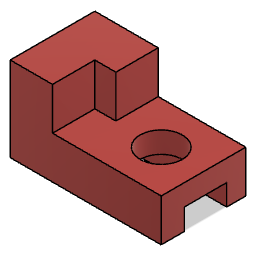
3d14 v1 (Autodesk Fusion 360 design; units mm, degrees)
Autodesk Fusion 360 part; units mm, degrees
sketch "Sketch1" plane through (0, 0, 0) normal (0, 0, 1) x (1, 0, 0)
  line L0 (0, 0) -> (0, 28)
  line L1 (0, 28) -> (14, 28)
  line L2 (14, 28) -> (14, 14)
  line L3 (14, 14) -> (50, 14)
  line L4 (50, 14) -> (50, 0)
  line L5 (50, 0) -> (0, 0)
  dimension "d1" = 14
  dimension "d2" = 14
  dimension "d3" = 14
  dimension "d4" = 50
  constraint coincident L0.start L5.end
  constraint vertical L0
  constraint perpendicular L0 L1
  constraint perpendicular L1 L2
  constraint perpendicular L0 L3
  constraint perpendicular L1 L4
  constraint perpendicular L0 L5
  measures "d1" distance of L3.end L4.end
  measures "d2" distance of L1.end L2.end
  measures "d3" distance of L0.end L1.end
  measures "d4" distance of L0.start L4
extrude "Extrude1" add sketch "Sketch1" along normal mid plane 28
sketch "Sketch2" plane through (0, 0, 0) normal (0, 0, 1) x (1, 0, 0)
  line L0 (14, 28) -> (21, 28)
  line L1 (21, 28) -> (21, 14)
  line L2 (21, 14) -> (14, 14)
  line L3 (14, 14) -> (14, 28)
  point P0 (14, 28)
  point P1 (14, 14)
  dimension "d7" = 7
  dimension "d8" = 14
  constraint horizontal L0
  constraint vertical L1
  constraint horizontal L2
  constraint vertical L3
  constraint vertical P0 L0.start
  constraint coincident P1 L2.end
  measures "d7" distance of P0 L0.end
  measures "d8" distance of P0 L2.end
extrude "Extrude2" add sketch "Sketch2" against normal blind 14
sketch "Sketch3" plane through (50, 0, 0) normal (1, 0, 0) x (0, 0, -1)
  line L0 (14, 14) -> (-14, 14)
  line L1 (-14, 14) -> (-14, 0)
  line L2 (-14, 0) -> (14, 0)
  line L3 (14, 0) -> (14, 14)
  line L4 (-6.3263, 0) -> (-6.3263, 7)
  line L5 (-6.3263, 7) -> (7.6737, 7)
  line L6 (7.6737, 7) -> (7.6737, 0)
  line L7 (0, 18) -> (0, 0) construction
  line L8 (0, 0) -> (0, -4) construction
  dimension "d11" = 14
  dimension "d12" = 14
  dimension "d13" = 14
  dimension "d14" = 7.6737
  dimension "d15" = 90
  dimension "d16" = 7
  constraint coincident L2 L4.start
  constraint perpendicular L2 L4
  constraint perpendicular L4 L5
  constraint coincident L2 L6.end
  constraint perpendicular L2 L6
  constraint vertical L7
  constraint coincident L2 L7.end
  constraint vertical L8
  measures "d11" distance of L4.start L6.end
  measures "d12" distance of L2.end L7.end
  measures "d13" distance of L4.end L5.end
  measures "d14" distance of L1.end L4
  measures "d15" angle of L1 L5
  measures "d16" distance of L2 L5
extrude "Extrude3" cut sketch "Sketch3" against normal blind 50 contours L2 L4 L5 L6
sketch "Sketch4" plane through (0, 14, 0) normal (0, 1, 0) x (-1, 0, 0)
  line L0 (-21, -14) -> (-21, 0)
  line L1 (-21, 0) -> (-14, 0)
  line L2 (-14, 0) -> (-14, 14)
  line L3 (-14, 14) -> (-50, 14)
  line L4 (-50, 14) -> (-50, -14)
  line L5 (-50, -14) -> (-21, -14)
  line L6 (5.2801, -7) -> (-65, -7) construction
  line L7 (5, 7) -> (-62.1492, 7) construction
  circle A0 centre (-36, 0) radius 7
  dimension "d19" = 7
  dimension "d20" = 7
  dimension "d21" = 14
  dimension "d22" = 14
  constraint perpendicular L0 L6
  constraint horizontal L7
  measures "d19" distance of L5 L6
  measures "d20" distance of L3 L7
  measures "d21" diameter of A0
  measures "d22" horizontal distance of L3.end A0.centre
extrude "Extrude4" cut sketch "Sketch4" against normal blind 7 contours A0
